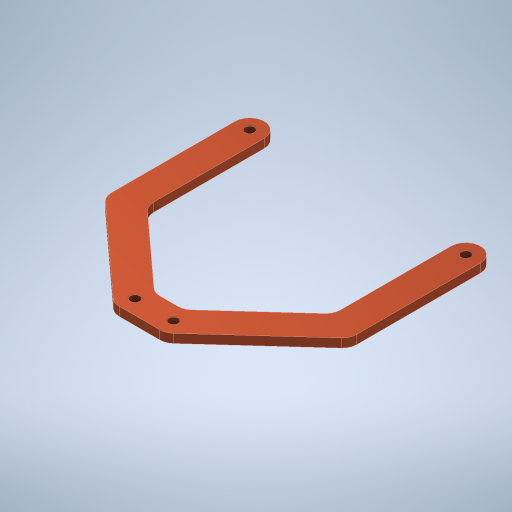
# Autodesk Inventor part: Claw4
Saved by Autodesk Inventor 2024 (Build 280153000, 153)
## iProperties
Created: 2022-11-29
Part Number: Claw4
Material: Copper, Cast
Document SubType Name: Modeling
Designer: kakik
Density: 8.94 g/cm^3
Appearance: Copper - Satin
Author: kakik
Autodesk Inventor part; units mm, degrees
ref_plane "YZ Plane" through (0, 0, 0) normal (1, 0, 0) x (0, 1, 0)
ref_plane "XZ Plane" through (0, 0, 0) normal (0, 1, 0) x (-1, 0, 0)
ref_plane "XY Plane" through (0, 0, 0) normal (0, 0, 1) x (1, 0, 0)
sketch "Sketch3" plane through (0, 0, 0) normal (0, 1, 0) x (-1, 0, 0)
  line L0 (0, 0) -> (5, 0)
  line L1 (31.8661, -24.4237) -> (31.8661, -64.4237)
  line L2 (41.8661, -64.4237) -> (41.8661, -20)
  line L3 (0, 10) -> (0, 0)
  line L4 (8.8661, 10) -> (41.8661, -20)
  line L5 (31.8661, -24.4237) -> (5, 0)
  line L6 (8.8661, 10) -> (0, 10)
  line L7 (5, 0) -> (0, 0)
  line L8 (31.8661, -24.4237) -> (31.8661, -64.4237)
  line L9 (41.8661, -64.4237) -> (41.8661, -20)
  line L10 (5, 0) -> (0, 0)
  arc A0 (31.8661, -64.4237) -> (41.8661, -64.4237) centre (36.8661, -64.4237) ccw
  circle A1 centre (0, -35.9984) radius 30
  point P0 (31.8661, -44.4237)
  point P1 (0, 5)
  dimension "d51" = 10
  dimension "d56" = 10
  dimension "d57" = 30
  dimension "d58" = 33
  dimension "d59" = 5
  dimension "d60" = 5
  dimension "d61" = 40
  dimension "d64" = 10
  dimension "d65" = 10
  dimension "d66" = 60
  constraints: 22 end point, 3 perpendicular, 2 centre point, 2 midpoint, 2 point on circle, 1 collinear, 1 horizontal, 1 horizontal alignment, 1 parallel, 1 tangent, 1 vertical alignment
  measures "d51" distance of L3.start L0.start
  measures "d56" distance between parallel lines of L5 L4
  measures "d57" vertical distance of L4.start L2.end
  measures "d58" horizontal distance of L4.start L2.end
  measures "d59" radius of A0
  measures "d60" distance of L0.start L0.end
  measures "d61" distance of L1.start L1.end
  measures "d64" distance from line of point (31.866, -44.424) L2
  measures "d65" vertical distance of L4.start L0.end
  measures "d66" diameter of A1
extrude "Extrusion2" add sketch "Sketch3" along normal blind 3 contours L3 L6 L4 L2 A0 L1 L5 L0
sketch "Sketch4" plane through (0, 3, 0) normal (0, 1, 0) x (1, 0, 0)
  line L0 (0, -10) -> (0, 0) projected
  arc A0 (-31.8661, 64.4237) -> (-41.8661, 64.4237) centre (-36.8661, 64.4237) ccw projected
  point P0 (-6.55, -5)
  point P1 (0, -5)
  point P2 (-36.8661, 69.4237)
  dimension "d77" = 6.55
  constraints: 2 horizontal alignment, 1 midpoint, 1 point on circle, 1 vertical alignment
  measures "d77" distance from line of L0 point (-6.55, -5)
hole "Hole2" at (-6.55, 3, 5) at (-36.8661, 3, -64.4237) direction (0, -1, 0) diameter 3.2 end through all clearance for "Countersunk Flat Head Screw DIN EN ISO 2009" size "M3" standard "DIN"
fillet "Fillet1" radius 5 4 edges at (-8.8661, 1.5, 10) (-41.8661, 1.5, -20) (-31.8661, 1.5, -24.4237) (-5, 1.5, 0)
mirror "Mirror3" about plane through (0, 0, 10) normal (1, 0, 0) of "Extrusion2", "Hole2", "Fillet1"
body "Solid2"
